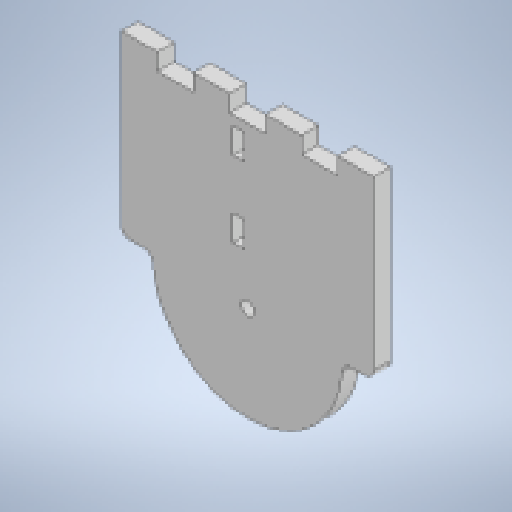
# Autodesk Inventor part: wheel1
Saved by Autodesk Inventor 2023.1 (Build 271208000, 208)
## iProperties
Created: 2023-03-14
Part Number: wheel1
Material: Типовые
Document SubType Name: Modeling
Designer: User
Density: 1 g/cm^3
Appearance: По умолчанию
Author: User
Autodesk Inventor part; units mm, degrees
ref_plane "YZ Plane" through (0, 0, 0) normal (1, 0, 0) x (0, 1, 0)
ref_plane "XZ Plane" through (0, 0, 0) normal (0, 1, 0) x (-1, 0, 0)
ref_plane "РабПлоскость1" through (-34.9448, 28.465, -130.3508) normal (0, 0, 1) x (1, 0, 0)
sketch "Эскиз1" plane through (-34.9448, 28.465, -130.3508) normal (0, 0, 1) x (1, 0, 0)
  line L0 (0, 3.6904) -> (-12.8571, 3.6904) construction
  line L1 (0, 3.6904) -> (0, 9.6905) projected
  line L2 (-12.8571, 9.6905) -> (0, 9.6905) projected
  line L3 (-12.8571, 3.6904) -> (-12.8571, 9.6905)
  line L4 (25.7143, 3.6904) -> (12.8571, 3.6904) construction
  line L5 (25.7143, 3.6904) -> (25.7143, 9.6905) projected
  line L6 (12.8571, 9.6905) -> (25.7143, 9.6905) projected
  line L7 (12.8571, 3.6904) -> (12.8571, 9.6905)
  line L8 (51.4286, 3.6904) -> (38.5714, 3.6904) construction
  line L9 (51.4286, 3.6904) -> (51.4286, 9.6905) projected
  line L10 (38.5714, 9.6905) -> (51.4286, 9.6905) projected
  line L11 (38.5714, 3.6904) -> (38.5714, 9.6905)
  line L12 (77.1429, 3.6904) -> (64.2857, 3.6904) construction
  line L13 (77.1429, 3.6904) -> (77.1429, 9.6905) projected
  line L14 (64.2857, 9.6905) -> (77.1429, 9.6905) projected
  line L15 (64.2857, 3.6904) -> (64.2857, 9.6905)
  line L16 (0, 3.6904) -> (12.8571, 3.6904)
  line L17 (25.7143, 3.6904) -> (38.5714, 3.6904)
  line L18 (51.4286, 3.6904) -> (64.2857, 3.6904)
  line L19 (-12.8571, 3.6904) -> (-12.8571, -50.3096)
  line L20 (-9.8571, -53.3096) -> (-4.7353, -53.3096)
  line L21 (77.1429, 3.6904) -> (77.1429, -50.3096)
  line L22 (74.1429, -53.3096) -> (69.021, -53.3096)
  line L23 (-1.8571, -53.3096) -> (66.1429, -53.3096) construction
  arc A0 (-1.7452, -56.0663) -> (66.0309, -56.0663) centre (32.1429, -53.3096) ccw
  arc A1 (-1.7452, -56.0663) -> (-4.7353, -53.3096) centre (-4.7353, -56.3096) ccw
  arc A2 (69.021, -53.3096) -> (66.0309, -56.0663) centre (69.021, -56.3096) ccw
  arc A3 (74.1429, -53.3096) -> (77.1429, -50.3096) centre (74.1429, -50.3096) ccw
  arc A4 (-12.8571, -50.3096) -> (-9.8571, -53.3096) centre (-9.8571, -50.3096) ccw
  circle A5 centre (32.1429, -53.3095) radius 2.375
  point P0 (34.9448, -28.465)
  point P1 (77.1429, -53.3096)
  dimension "d0" = 57
  dimension "d1" = 34
  dimension "d2" = 3
  dimension "d3" = 6
  dimension "d14" = 4.75
  constraints: 24 end point, 12 point on circle, 8 tangent, 6 centre point, 4 collinear, 4 point on line, 3 equal radius, 2 perpendicular, 2 vertical, 1 horizontal, 1 horizontal alignment, 1 midpoint
  measures "d0" distance of L12.start point (77.143, -53.31)
  measures "d1" radius of A0
  measures "d2" radius of A1
  measures "d3" distance between parallel lines of L8 L10
  measures "d14" diameter of A5
ref_plane "РабПлоскость2" through (-162.802, 331.465, 111.3492) normal (0, 0, 1) x (1, 0, 0)
extrude "Выдавливание1" add sketch "Эскиз1" along normal blind 6
sketch "Эскиз6" plane through (-34.9448, 28.465, -130.3508) normal (0, 0, -1) x (-1, 0, 0)
  line L0 (-30.9731, -35.6894) -> (-30.9731, -26.6894)
  line L1 (-30.9731, -26.6894) -> (-26.9731, -26.6894)
  line L2 (-26.9731, -35.6894) -> (-30.9731, -35.6894)
  line L3 (-26.9731, -26.6894) -> (-26.9731, -35.6894)
  line L4 (-26.9731, 0.3106) -> (-26.9731, -8.6894)
  line L5 (-26.9731, -8.6894) -> (-30.9731, -8.6894)
  line L6 (-30.9731, 0.3106) -> (-26.9731, 0.3106)
  line L7 (-30.9731, -8.6894) -> (-30.9731, 0.3106)
  constraints: 16 end point
extrude "Выдавливание5" cut sketch "Эскиз6" against normal blind 10
sketch "Эскиз2" plane through (-34.9448, 28.465, -130.3508) normal (0, 0, -1) x (-1, 0, 0)
  line L0 (-4.9286, 3.6904) -> (-4.9286, -2.6596)
  line L1 (-4.9286, -2.6596) -> (-3.6786, -2.6596)
  line L2 (-3.6786, -2.6596) -> (-3.6786, -4.9596)
  line L3 (-3.6786, -4.9596) -> (-4.9286, -4.9596)
  line L4 (-4.9286, -4.9596) -> (-4.9286, -11.3096)
  line L5 (-4.9286, -11.3096) -> (-7.9286, -11.3096)
  line L6 (-7.9286, -11.3096) -> (-7.9286, -4.9596)
  line L7 (-7.9286, -4.9596) -> (-9.1786, -4.9596)
  line L8 (-9.1786, -4.9596) -> (-9.1786, -2.6596)
  line L9 (-9.1786, -2.6596) -> (-7.9286, -2.6596)
  line L10 (-7.9286, -2.6596) -> (-7.9286, 3.6904)
  line L11 (-56.3571, 3.6904) -> (-59.3571, 3.6904)
  line L12 (-56.3571, 3.6904) -> (-56.3571, -2.6596)
  line L13 (-56.3571, -2.6596) -> (-55.1071, -2.6596)
  line L14 (-55.1071, -2.6596) -> (-55.1071, -4.9596)
  line L15 (-55.1071, -4.9596) -> (-56.3571, -4.9596)
  line L16 (-56.3571, -4.9596) -> (-56.3571, -11.3096)
  line L17 (-56.3571, -11.3096) -> (-59.3571, -11.3096)
  line L18 (-59.3571, -11.3096) -> (-59.3571, -4.9596)
  line L19 (-59.3571, -4.9596) -> (-60.6071, -4.9596)
  line L20 (-60.6071, -4.9596) -> (-60.6071, -2.6596)
  line L21 (-60.6071, -2.6596) -> (-59.3571, -2.6596)
  line L22 (-59.3571, -2.6596) -> (-59.3571, 3.6904)
  line L23 (-56.3571, 3.6904) -> (-59.3571, 3.6904) projected
  line L24 (-4.9286, 3.6904) -> (-7.9286, 3.6904) projected
  line L25 (-25.7143, 3.6904) -> (-25.7143, 9.6905) projected
  line L26 (-38.5714, 3.6904) -> (-25.7143, 3.6904) projected
  line L27 (-38.5714, 9.6905) -> (-38.5714, 3.6904) projected
  line L28 (-51.4286, 3.6904) -> (-51.4286, 9.6905) projected
  line L29 (-64.2857, 3.6904) -> (-51.4286, 3.6904) projected
  line L30 (-64.2857, 9.6905) -> (-64.2857, 3.6904) projected
  line L31 (-77.1429, -50.3096) -> (-77.1429, 9.6905) projected
  arc A0 (-77.1429, -50.3096) -> (-74.1429, -53.3096) centre (-74.1429, -50.3096) ccw projected
  line L32 (-69.021, -53.3096) -> (-74.1429, -53.3096) projected
  arc A1 (-66.0309, -56.0663) -> (-69.021, -53.3096) centre (-69.021, -56.3096) ccw projected
  arc A2 (-66.0309, -56.0663) -> (1.7452, -56.0663) centre (-32.1429, -53.3096) ccw projected
  arc A3 (4.7353, -53.3096) -> (1.7452, -56.0663) centre (4.7353, -56.3096) ccw projected
  line L33 (9.8571, -53.3096) -> (4.7353, -53.3096) projected
  arc A4 (9.8571, -53.3096) -> (12.8571, -50.3096) centre (9.8571, -50.3096) ccw projected
  line L34 (12.8571, 9.6905) -> (12.8571, -50.3096) projected
  line L35 (0, 3.6904) -> (0, 9.6905) projected
  line L36 (-12.8571, 3.6904) -> (0, 3.6904) projected
  line L37 (-12.8571, 9.6905) -> (-12.8571, 3.6904) projected
  circle A5 centre (-32.1429, -53.3095) radius 2.375 projected
  line L38 (-25.7143, 9.6905) -> (-12.8571, 9.6905) projected
  line L39 (-51.4286, 9.6905) -> (-38.5714, 9.6905) projected
  line L40 (-77.1429, 9.6905) -> (-64.2857, 9.6905) projected
  line L41 (0, 9.6905) -> (12.8571, 9.6905) projected
  point P0 (-6.4286, 0)
  constraints: 46 end point, 14 perpendicular, 14 point on line, 7 equal length, 2 vertical
sketch "Эскиз4" plane through (29.3409, 38.1554, -130.3508) normal (0, 1, 0) x (1, 0, 0)
  line L0 (-77.1429, 0) -> (-77.1429, -6) projected
  line L1 (12.8571, 0) -> (-77.1429, 0)
  line L2 (-77.1429, 0) -> (-77.1429, -6)
  line L3 (-77.1429, -6) -> (12.8571, -6)
  line L4 (12.8571, -6) -> (12.8571, 0)
  point P0 (-29.3409, -130.3508)
  constraints: 8 end point, 2 parallel, 1 horizontal, 1 perpendicular
sketch "Эскиз5" plane through (-34.9448, 28.465, -130.3508) normal (0, 0, -1) x (-1, 0, 0)
  line L0 (-236.4804, 8.6905) -> (-77.1429, 8.6905) construction
  line L1 (-77.1429, 8.6905) -> (-64.2857, 8.6905) construction
  line L2 (-64.2857, 8.6905) -> (-51.4286, 8.6905) construction
  line L3 (-51.4286, 8.6905) -> (-38.5714, 8.6905) construction
  line L4 (-38.5714, 8.6905) -> (-25.7143, 8.6905) construction
  line L5 (-25.7143, 8.6905) -> (-12.8571, 8.6905) construction
  line L6 (-12.8571, 8.6905) -> (0, 8.6905) construction
  line L7 (0, 8.6905) -> (12.8571, 8.6905) construction
  line L8 (12.8571, 8.6905) -> (44.8254, 8.6905) construction
  line L9 (44.8254, 8.6905) -> (44.8254, 3.6905) construction
  line L10 (44.8254, 3.6905) -> (12.8571, 3.6905) construction
  line L11 (12.8571, 3.6905) -> (12.8571, 8.6905) construction
  line L12 (-236.4804, 3.6905) -> (-236.4804, 8.6905) construction
  line L13 (-77.1429, 3.6905) -> (-236.4804, 3.6905) construction
  line L14 (-64.2857, 3.6905) -> (-77.1429, 3.6905) construction
  line L15 (-51.4286, 3.6905) -> (-64.2857, 3.6905) construction
  line L16 (-38.5714, 3.6905) -> (-51.4286, 3.6905) construction
  line L17 (-25.7143, 3.6905) -> (-38.5714, 3.6905) construction
  line L18 (-12.8571, 3.6905) -> (-25.7143, 3.6905) construction
  line L19 (0, 3.6905) -> (-12.8571, 3.6905) construction
  line L20 (12.8571, 3.6905) -> (0, 3.6905) construction
  line L21 (-77.1429, 8.6905) -> (-77.1429, 3.6905) construction
  line L22 (-64.2857, 3.6905) -> (-64.2857, 8.6905) construction
  line L23 (-51.4286, 8.6905) -> (-51.4286, 3.6905) construction
  line L24 (-38.5714, 3.6905) -> (-38.5714, 8.6905) construction
  line L25 (-25.7143, 8.6905) -> (-25.7143, 3.6905) construction
  line L26 (-12.8571, 3.6905) -> (-12.8571, 8.6905) construction
  line L27 (0, 8.6905) -> (0, 3.6905) construction
  line L28 (-242.4804, 3.6905) -> (-352.8338, 3.6905) construction
  line L29 (-352.8338, 3.6905) -> (-352.8338, 8.6905) construction
  line L30 (-352.8338, 8.6905) -> (-242.4804, 8.6905) construction
  line L31 (-242.4804, 8.6905) -> (-242.4804, 3.6905) construction
  line L32 (-34.1429, 3.6915) -> (-30.1429, 3.6915) construction
  line L33 (-30.1429, -50.9345) -> (-34.1429, -50.9345) construction
  line L34 (-34.1429, 3.6915) -> (-30.1429, -50.9345) construction
  line L35 (-30.1429, 3.6915) -> (-34.1429, -50.9345) construction
  circle A0 centre (-32.1429, -53.3095) radius 2.375 construction
  line L36 (-34.1429, -5.6215) -> (-30.1429, -5.6215)
  line L37 (-30.1429, -41.6215) -> (-34.1429, -41.6215)
  line L38 (-34.1429, -5.6215) -> (-30.1429, -41.6215) construction
  line L39 (-30.1429, -5.6215) -> (-34.1429, -41.6215) construction
  line L40 (-34.1429, -14.6215) -> (-30.1429, -14.6215)
  line L41 (-30.1429, -32.6215) -> (-34.1429, -32.6215)
  line L42 (-34.1429, -14.6215) -> (-30.1429, -32.6215) construction
  line L43 (-30.1429, -14.6215) -> (-34.1429, -32.6215) construction
  line L44 (-34.1429, -41.6215) -> (-34.1429, -32.6215)
  line L45 (-34.1429, -14.6215) -> (-34.1429, -5.6215)
  line L46 (-30.1429, -5.6215) -> (-30.1429, -14.6215)
  line L47 (-30.1429, -32.6215) -> (-30.1429, -41.6215)
  line L48 (-30.1429, -32.6215) -> (-30.1429, -41.6215) construction
  line L49 (-34.1429, -50.9345) -> (-34.1429, -32.6215) construction
  line L50 (-34.1429, -14.6215) -> (-34.1429, 3.6915) construction
  line L51 (-30.1429, 3.6915) -> (-30.1429, 3.6905) construction
  line L52 (-30.1429, -5.6215) -> (-30.1429, -14.6215) construction
  point P0 (-34.9448, -28.465)
  point P1 (-32.1429, -23.6215)
  point P2 (-32.1429, -50.9345)
  dimension "d20" = 4
  dimension "d21" = 54.626
  constraints: 106 end point, 23 horizontal, 12 parallel, 12 vertical, 7 midpoint, 5 perpendicular, 1 point on line, 1 vertical alignment, 25 other
  measures "d20" distance of L33.start L33.end
  measures "d21" distance of L32.end L33.start
equation "\"d4\" = d3"
